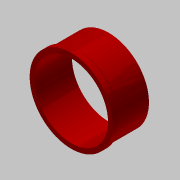
# Autodesk Inventor part: A1-19037-100-06 HCWI liner - pup - as cast
Saved by Autodesk Inventor 2017.3 (Build 213257000, 257)
## iProperties
Created: 2019-08-22
Part Number: A1-19037-100-06 HCWI liner - pup - as cast
Material: Iron, HCWI
Document SubType Name: Modeling
Designer: GVD
Density: 7.33517 g/cm^3
Appearance: Iron Gray(1)
Project: A1-19037--CNUL Albian CST laterals
Mass: 189760 g
Surface Area: 17053.4 cm^2
Volume: 25869.9 cm^3
Description: 26 1/2" ID x 1 1/4" WALL x 12 1/2" HCWI LINER, ASTM A532 CLASS III TYPE A, PF# 503368
Constructed By: Graeme_Van_Dongen
Project Name: CST laterals
Author: GVD
Autodesk Inventor part; units mm, degrees
ref_plane "YZ Plane" through (0, 0, 0) normal (1, 0, 0) x (0, 1, 0)
ref_plane "XZ Plane" through (0, 0, 0) normal (0, 1, 0) x (-1, 0, 0)
ref_plane "XY Plane" through (0, 0, 0) normal (0, 0, 1) x (1, 0, 0)
sketch "Sketch1" plane through (0, 0, 0) normal (0, 0, 1) x (1, 0, 0)
  circle A0 centre (0, 0) radius 336.55
  circle A1 centre (0, 0) radius 368.3
  dimension "d0" = 673.1
  dimension "d1" = 736.6
  constraints: 2 centre point, 2 coincident
  measures "d0" diameter of A0
  measures "d1" diameter of A1
extrude "Extrusion1" add sketch "Sketch1" along normal blind 304.8
sketch "Sketch2" plane through (0, 0, 304.8) normal (0, 0, 1) x (1, 0, 0)
  circle A0 centre (0, 0) radius 368.3 projected
  circle A1 centre (0, 0) radius 371.221
  circle A2 centre (0, 0) radius 374.396
  dimension "d4" = 742.442
  dimension "d5" = 748.792
  constraints: 2 centre point, 2 coincident
  measures "d4" diameter of A1
  measures "d5" diameter of A2
extrude "Extrusion2" add sketch "Sketch2" against normal blind 50.8 contours A1
extrude "Extrusion3" add sketch "Sketch2" against normal blind 25.4 contours A2
chamfer "Chamfer1" distance 2.921 angle 45 1 edges at (-368.3, 0, 254)
sketch "Sketch3" plane through (0, 0, 0) normal (0, 0, -1) x (-1, 0, 0)
  circle A0 centre (0, 0) radius 355.346
  circle A1 centre (0, 0) radius 336.55 projected
  dimension "d13" = 710.692
  constraints: 1 centre point, 1 coincident
  measures "d13" diameter of A0
extrude "Extrusion4" add sketch "Sketch3" along normal blind 12.7
fillet "Fillet1" radius 0.7937 2 edges at (355.346, 0, 0) (-371.221, 0, 279.4)
chamfer "Chamfer2" distance 0.7937 angle 45 1 edges at (355.346, 0, -12.7)
chamfer "Chamfer3" distance 0.7937 angle 45 1 edges at (-374.396, 0, 279.4)
sketch "Sketch4" plane through (0, 0, 0) normal (1, 0, 0) x (0, 1, 0)
  line L0 (371.221, 278.6063) -> (371.221, 254) construction
  line L1 (-374.396, 304.8) -> (374.396, 304.8) construction
  line L2 (371.221, 273.05) -> (369.4409, 271.2699)
  arc A0 (369.4409, 271.2699) -> (368.046, 267.9023) centre (372.8085, 267.9023) ccw
  line L3 (368.046, 267.9023) -> (368.046, 267.0852)
  arc A1 (368.046, 267.0852) -> (369.4409, 263.7176) centre (372.8085, 267.0852) ccw
  line L4 (369.4409, 263.7176) -> (371.221, 261.9375)
  line L5 (371.221, 261.9375) -> (371.221, 273.05)
  line L6 (0, -76.2) -> (0, 368.3) projected
  point P0 (0, 0)
  dimension "d23" = 11.1125
  dimension "d24" = 3.175
  dimension "d25" = 4.7625
  dimension "d26" = 31.75
  dimension "d27" = 45
  constraints: 8 end point, 4 point on circle, 4 tangent, 2 centre point, 2 point on line, 1 collinear, 1 equal radius, 1 perpendicular, 1 vertical
  measures "d23" distance of L2.start L4.end
  measures "d24" distance between parallel lines of L5 L3
  measures "d25" radius of A1
  measures "d26" distance from line of L1 L2.start
  measures "d27" angle of L5 L4
revolve "Revolution1" cut sketch "Sketch4" angle 360 about axis through (0, 0, -10) along (0, 0, 1)
sketch "Sketch5" plane through (0, 0, -12.7) normal (0, 0, -1) x (-1, 0, 0)
  circle A0 centre (0, 0) radius 336.55 projected
  circle A1 centre (0, 0) radius 368.3 projected
extrude "Extrusion5" add sketch "Sketch5" along normal blind 12.7 and the other way blind 12.7
sketch "Sketch6" plane through (0, 0, 304.8) normal (0, 0, 1) x (1, 0, 0)
  circle A0 centre (0, 0) radius 374.396 projected
  circle A1 centre (0, 0) radius 336.55 projected
  circle A2 centre (0, 0) radius 380.746
  dimension "d33" = 6.35
  constraints: 1 centre point
  measures "d33" radial gap between concentric circles of A0 A2
extrude "Extrusion6" add sketch "Sketch6" along normal blind 12.7 and the other way blind 50.8 contours A0 | A2
chamfer "Chamfer6" distance 9.525 angle 45 1 edges at (-380.746, 0, 254)
equation "\"d10\" = -0.5 * d1 + 0.5 * d4"
body "Solid1"
